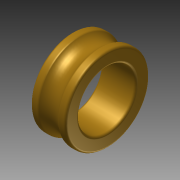
# Autodesk Inventor part: InelInterior
Saved by Autodesk Inventor 2011 SP2 (Build 150309200, 309)
## iProperties
Created: 2023-03-13
Part Number: InelInterior
Document SubType Name: Modeling
Designer: utilizator
Density: 1 g/cm^3
Author: utilizator
Autodesk Inventor part; units mm, degrees
ref_plane "YZ Plane" through (0, 0, 0) normal (1, 0, 0) x (0, 1, 0)
ref_plane "XZ Plane" through (0, 0, 0) normal (0, 1, 0) x (-1, 0, 0)
ref_plane "XY Plane" through (0, 0, 0) normal (0, 0, 1) x (1, 0, 0)
sketch "Sketch1" plane through (0, 0, 0) normal (0, 0, 1) x (1, 0, 0)
  line L0 (0, -9) -> (0, 54) projected
  line L1 (-21.7, 0) -> (21.7, 0) projected
  line L2 (-15.5, 37) -> (15.5, 37) construction
  line L3 (15.5, 37) -> (15.5, 25)
  line L4 (15.5, 25) -> (-15.5, 25)
  line L5 (-15.5, 25) -> (-15.5, 37)
  arc A0 (-8.9443, 37) -> (8.9443, 37) centre (0, 45) ccw
  line L6 (-15.5, 37) -> (-8.9443, 37)
  line L7 (8.9443, 37) -> (15.5, 37)
  point P0 (0, 0)
  point P1 (0, 37)
  dimension "d0" = 31
  dimension "d1" = 37
  dimension "d2" = 25
  dimension "d3" = 12
  dimension "d4" = 8
  constraints: 12 end point, 2 collinear, 2 parallel, 2 point on circle, 2 point on line, 2 vertical alignment, 1 centre point, 1 horizontal, 1 midpoint, 1 perpendicular
  measures "d0" distance of L3.end L4.end
  measures "d1" distance of point (0, 0) point (0, 37)
  measures "d2" distance from line of point (0, 0) L4
  measures "d3" radius of A0
  measures "d4" distance from line of L2 A0.centre
revolve "Revolution1" add sketch "Sketch1" angle 360 about axis through (-10, 0, 0) along (1, 0, 0)
fillet "Fillet1" radius 2 6 edges at (15.5, -37, 0) (8.9443, -37, 0) (-8.9443, -37, 0) (-15.5, -37, 0) (15.5, -25, 0) (-15.5, -25, 0)
body "Solid1"
